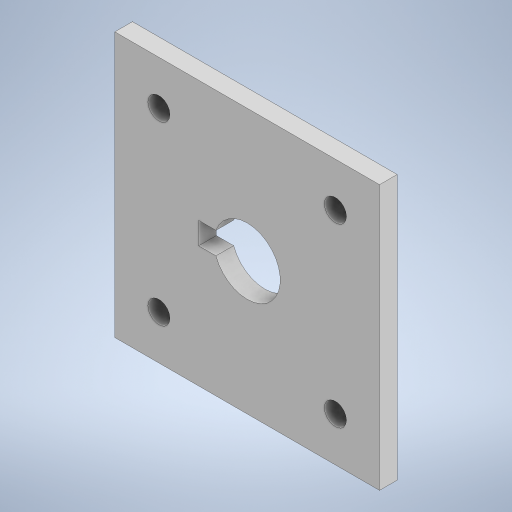
# Autodesk Inventor part: FlanschV1
Saved by Autodesk Inventor 2024.4 (Build 284460000, 460)
## iProperties
Created: 2025-11-05
Part Number: FlanschV1
Material: Generic
Document SubType Name: Modeling
Designer: jonas
Density: 1 g/cm^3
Appearance: Default
Author: jonas
Autodesk Inventor part; units mm, degrees
ref_plane "YZ Plane" through (0, 0, 0) normal (1, 0, 0) x (0, 1, 0)
ref_plane "XZ Plane" through (0, 0, 0) normal (0, 1, 0) x (-1, 0, 0)
ref_plane "XY Plane" through (0, 0, 0) normal (0, 0, 1) x (1, 0, 0)
sketch "Sketch1" plane through (0, 0, 0) normal (0, 1, 0) x (-1, 0, 0)
  line L0 (0, 11.1111) -> (0, -11.1111) construction
  line L1 (-5.5895, 0) -> (5.5895, 0) construction
  line L2 (30, 30) -> (-30, 30)
  line L3 (-30, 30) -> (-30, -30)
  line L4 (-30, -30) -> (30, -30)
  line L5 (30, -30) -> (30, 30)
  arc A0 (7.0711, 2.5) -> (7.0711, -2.5) centre (0, 0) ccw
  line L6 (7.0711, 2.5) -> (11, 2.5)
  line L7 (11, 2.5) -> (11, -2.5)
  line L8 (11, -2.5) -> (7.0711, -2.5)
  dimension "d0" = 60
  dimension "d1" = 15
  dimension "d2" = 5
  dimension "d4" = 11
  constraints: 18 end point, 3 horizontal, 3 parallel, 3 perpendicular, 2 coincident, 2 midpoint, 2 point on circle, 1 centre point, 1 vertical, 3 other
  measures "d0" distance of L4.end L2.start
  measures "d1" diameter of A0
  measures "d2" distance of L6.end L7.end
  measures "d4" distance from line of point (0, 0) L7
extrude "Extrusion1" add sketch "Sketch1" along normal blind 4
sketch "Sketch2" plane through (0, 4, 0) normal (0, 1, 0) x (1, 0, 0)
  line L0 (-30, -30) -> (30, -30) projected
  line L1 (30, -30) -> (30, 30) projected
  line L2 (30, 30) -> (-30, 30) projected
  line L3 (-30, 30) -> (-30, -30) projected
  point P0 (0, 0)
  point P1 (-20, -20)
  point P2 (20, -20)
  point P3 (20, 20)
  point P4 (-20, 20)
  dimension "d7" = 10
  dimension "d8" = 10
  dimension "d9" = 10
  dimension "d10" = 10
  constraints: 2 horizontal alignment, 2 vertical alignment
  measures "d7" distance from line of L0 point (-20, -20)
  measures "d8" distance from line of L1 point (20, -20)
  measures "d9" distance from line of L2 point (20, 20)
  measures "d10" distance from line of L3 point (-20, 20)
hole "Hole1" at (-20, 4, 20) at (20, 4, 20) at (20, 4, -20) at (-20, 4, -20) direction (0, -1, 0) diameter 5 end through all
body "Solid1"
